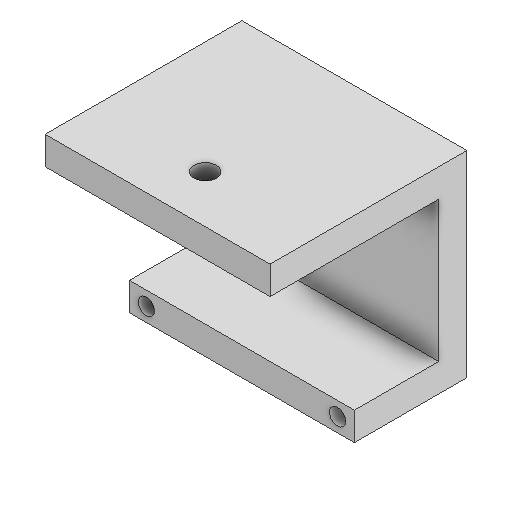
# Autodesk Inventor part: zacisk
Saved by Autodesk Inventor 2025.1 (Build 291241000, 241)
## iProperties
Created: 2025-05-14
Part Number: zacisk
Material: Ogólny
Document SubType Name: Modeling
Designer: Maciej
Density: 1 g/cm^3
Appearance: Domyślna
Author: Maciej
Autodesk Inventor part; units mm, degrees
ref_plane "YZ Plane" through (0, 0, 0) normal (1, 0, 0) x (0, 1, 0)
ref_plane "XZ Plane" through (0, 0, 0) normal (0, 1, 0) x (-1, 0, 0)
ref_plane "XY Plane" through (0, 0, 0) normal (0, 0, 1) x (1, 0, 0)
sketch "Szkic1" plane through (0, 0, 0) normal (0, 0, 1) x (1, 0, 0)
  line L0 (0, 0) -> (40, 0)
  line L1 (40, 0) -> (40, 30)
  line L2 (40, 30) -> (0, 30)
  line L3 (0, 30) -> (0, 0)
  dimension "d0" = 40
  dimension "d1" = 30
  constraints: 8 end point, 3 perpendicular, 1 horizontal
  measures "d0" distance of L0.start L0.end
  measures "d1" distance of L0.end L1.end
extrude "Wyciągnięcie proste1" add sketch "Szkic1" along normal blind 5
sketch "Szkic2" plane through (0, 0, 5) normal (0, 0, 1) x (1, 0, 0)
  line L0 (40, 30) -> (0, 30) projected
  line L1 (0, 30) -> (40, 30)
  line L2 (40, 30) -> (40, 25)
  line L3 (40, 25) -> (0, 25)
  line L4 (0, 30) -> (0, 0) projected
  dimension "d4" = 5
  constraints: 6 end point, 2 perpendicular, 1 collinear, 1 point on line
  measures "d4" distance of L0.start L2.end
extrude "Wyciągnięcie proste2" add sketch "Szkic2" along normal blind 30
sketch "Szkic5" plane through (0, 0, 0) normal (0, 0, -1) x (-1, 0, 0)
  line L0 (-40, 0) -> (-40, 25) projected
  line L1 (-40, 0) -> (0, 0)
  line L2 (0, 0) -> (0, -5)
  line L3 (0, -5) -> (-40, -5)
  line L4 (-40, -5) -> (-40, 0)
  dimension "d7" = 5
  constraints: 8 end point, 3 perpendicular, 1 horizontal
  measures "d7" distance of L1.end L2.end
extrude "Wyciągnięcie proste3" add sketch "Szkic5" against normal blind 20
sketch "Szkic6" plane through (0, 25, 5) normal (0, -1, 0) x (1, 0, 0)
  point P0 (0, -5)
  point P1 (20, 21.543)
hole "Otwór1" at (20, 25, 26.543) direction (0, 1, 0) diameter 4 end through all clearance for "Śruba ze łbem płaskim obrobiona" size "M4" standard "ANSI Profil metryczny M"
sketch "Szkic7" plane through (0, 25, 5) normal (0, -1, 0) x (1, 0, 0)
  circle A0 centre (20, 21.543) radius 2 projected
  circle A1 centre (20, 21.543) radius 3
  point P0 (0, -5)
  dimension "d17" = 6
  constraints: 1 centre point, 1 coincident
  measures "d17" diameter of A1
extrude "Wyciągnięcie proste4" cut sketch "Szkic7" against normal blind 2 contours A0 | A1
sketch "Szkic8" plane through (0, 0, 0) normal (0, 0, -1) x (-1, 0, 0)
  line L0 (-40, -5) -> (-40, 30) projected
  line L1 (0, 30) -> (0, -5) projected
  point P0 (0, 0)
  point P1 (-37, -2.5)
  point P2 (-3, -2.5)
  dimension "d20" = 3
  dimension "d21" = 3
  measures "d20" distance from line of L0 point (-37, -2.5)
  measures "d21" distance from line of L1 point (-3, -2.5)
hole "Otwór2" at (37, -2.5, 0) at (3, -2.5, 0) direction (0, 0, 1) diameter 2.9 end through all clearance for "Śruba ze łbem płaskim obrobiona" size "M2.5" standard "ANSI Profil metryczny M"
equation "\"d21\" = d20"
